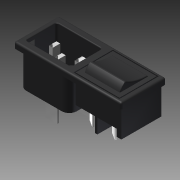
# Autodesk Inventor part: BZM27-Z0000-57B
Saved by Autodesk Inventor 2015 (Build 190159000, 159)
## iProperties
Created: 2013-06-08
Part Number: BZM27-Z0000-57B
Document SubType Name: Modeling
Designer: Estacion4
Density: 1 g/cm^3
Mass: 14.532 g
Surface Area: 93.949 cm^2
Volume: 14.532 cm^3
Material: Generic
Appearance: Rubber - Black - Version 1.1
Author: Estacion4
Autodesk Inventor part; units mm, degrees
ref_plane "YZ Plane" through (0, 0, 0) normal (1, 0, 0) x (0, 1, 0)
ref_plane "XZ Plane" through (0, 0, 0) normal (0, 1, 0) x (-1, 0, 0)
ref_plane "XY Plane" through (0, 0, 0) normal (0, 0, 1) x (1, 0, 0)
sketch "Boceto1" plane through (0, 0, 0) normal (0, 0, 1) x (1, 0, 0)
  line L0 (-28.75, 12) -> (28.75, 12)
  line L1 (28.75, 12) -> (28.75, -12)
  line L2 (28.75, -12) -> (-28.75, -12)
  line L3 (-28.75, -12) -> (-28.75, 12)
  line L4 (-27.45, 10.65) -> (27.45, 10.65)
  line L5 (27.45, 10.65) -> (27.45, -10.65)
  line L6 (27.45, -10.65) -> (-27.45, -10.65)
  line L7 (-27.45, -10.65) -> (-27.45, 10.65)
  point P0 (0, 0)
  point P1 (0, 12)
  point P2 (-28.75, 0)
  point P3 (-27.45, 0)
  point P4 (0, 10.65)
  dimension "d0" = 57.5
  dimension "d1" = 24
  dimension "d2" = 54.9
  dimension "d3" = 21.3
  constraints: 16 end point, 4 midpoint, 4 parallel, 2 horizontal, 2 horizontal alignment, 2 perpendicular, 2 vertical alignment
  measures "d0" distance of L0.start L0.end
  measures "d1" distance of L2.end L0.start
  measures "d2" distance of L4.start L4.end
  measures "d3" distance of L6.end L4.start
extrude "Extrusión1" add sketch "Boceto1" along normal blind 3.2 contours L0 L1 L2 L3 | L4 L5 L6 L7
sketch "Boceto2" plane through (0, 0, 0) normal (0, 0, -1) x (-1, 0, 0)
  line L0 (28.75, -12) -> (28.75, 12) projected
  line L1 (27.45, -10.65) -> (0.45, -10.65)
  line L2 (0.45, -10.65) -> (0.45, 10.65)
  line L3 (0.45, 10.65) -> (27.45, 10.65)
  line L4 (27.45, 10.65) -> (27.45, -10.65)
  line L5 (28.75, 12) -> (-28.75, 12) projected
  line L6 (-28.75, 12) -> (-28.75, -12) projected
  line L7 (-28.75, -12) -> (28.75, -12) projected
  line L8 (28.75, -12) -> (28.75, 12) projected
  point P0 (27.45, 0)
  point P1 (28.75, 0)
  point P2 (27.45, 0)
  dimension "d8" = 27
  dimension "d9" = 21.3
  constraints: 8 end point, 2 midpoint, 2 parallel, 1 coincident, 1 horizontal, 1 horizontal alignment, 1 perpendicular
  measures "d8" distance of L1.start L1.end
  measures "d9" distance of L3.end L1.start
extrude "Extrusión3" add sketch "Boceto2" along normal blind 17.8 contours L1 L2 L3 L4
fillet "Empalme1" radius 4 4 edges at (-27.45, -10.65, -8.9) (-27.45, 10.65, -8.9) (-0.45, 10.65, -8.9) (-0.45, -10.65, -8.9)
sketch "Boceto3" plane through (0, 0, 0) normal (0, 0, -1) x (-1, 0, 0)
  line L0 (-3.05, -10.65) -> (-27.45, -10.65)
  line L1 (-27.45, -10.65) -> (-27.45, 10.65)
  line L2 (-27.45, 10.65) -> (-3.05, 10.65)
  line L3 (-3.05, 10.65) -> (-3.05, -10.65)
  line L4 (-27.45, 10.65) -> (-27.45, -10.65) projected
  line L5 (-27.45, -10.65) -> (27.45, -10.65) projected
  line L6 (27.45, 10.65) -> (-27.45, 10.65) projected
  dimension "d13" = 24.4
  constraints: 8 end point, 2 parallel, 1 horizontal, 1 perpendicular
  measures "d13" distance between parallel lines of L1 L3
extrude "Extrusión4" add sketch "Boceto3" along normal blind 11.2
sketch "Boceto4" plane through (0, 0, -11.2) normal (0, 0, -1) x (-1, 0, 0)
  line L0 (-27.45, 10.65) -> (-3.05, 10.65) projected
  line L1 (-27.45, -10.65) -> (-27.45, 10.65) projected
  line L2 (-3.05, -10.65) -> (-27.45, -10.65) projected
  line L3 (-24.95, -10.65) -> (-24.95, 10.65)
  dimension "d16" = 2.5
  constraints: 2 end point, 2 point on line, 1 perpendicular
  measures "d16" distance between parallel lines of L1 L3
extrude "Extrusión5" add sketch "Boceto4" along normal blind 3.75
sketch "Boceto5" plane through (0, 0, -11.2) normal (0, 0, -1) x (-1, 0, 0)
  line L0 (-3.05, -10.65) -> (-24.95, -10.65) projected
  line L1 (-24.95, 10.65) -> (-3.05, 10.65) projected
  line L2 (-13.375, -10.65) -> (-14.625, -10.65)
  line L3 (-14.625, -10.65) -> (-14.625, 10.65)
  line L4 (-14.625, 10.65) -> (-13.375, 10.65)
  line L5 (-13.375, 10.65) -> (-13.375, -10.65)
  point P0 (-14, -10.65)
  dimension "d19" = 1.25
  constraints: 8 end point, 2 midpoint, 2 parallel, 2 point on line, 1 horizontal, 1 perpendicular
  measures "d19" distance between parallel lines of L3 L5
extrude "Extrusión6" add sketch "Boceto5" along normal blind 7.8
sketch "Boceto6" plane through (0, 0, -11.2) normal (0, 0, -1) x (-1, 0, 0)
  line L0 (-14.625, -10.65) -> (-14.625, 10.65) projected
  line L1 (-24.95, 10.65) -> (-14.625, 10.65) projected
  line L2 (-24.95, 10.65) -> (-24.95, -10.65) projected
  line L3 (-14.625, -10.65) -> (-24.95, -10.65) projected
  line L4 (-5.9821, -6.1326) -> (-9.9328, -8.6786)
  line L5 (-9.9328, -8.6786) -> (-10.3661, -8.0061)
  line L6 (-10.3661, -8.0061) -> (-6.4155, -5.4601)
  line L7 (-6.4155, -5.4601) -> (-5.9821, -6.1326)
  dimension "d22" = 0.8
  dimension "d23" = 4.7
  constraints: 8 end point, 2 parallel, 1 perpendicular
  measures "d22" distance between parallel lines of L6 L4
  measures "d23" distance of L4.start L4.end
extrude "Extrusión7" add sketch "Boceto6" along normal up to surface (7.8 mm away) contours L4 L5 L6 L7
pattern_linear "Patrón rectangular1" count 2 spacing 12 along (1, 0, 0) count 2 spacing 6 along (0, 1, 0) of "Extrusión7"
sketch "Boceto7" plane through (0, 0, -17.8) normal (0, 0, -1) x (-1, 0, 0)
  line L0 (27.45, 6.65) -> (27.45, -6.65) projected
  line L1 (4.45, 10.65) -> (23.45, 10.65) projected
  line L2 (17.1, -6.75) -> (10.8, -6.75)
  line L3 (10.8, -6.75) -> (10.8, -5.75)
  line L4 (10.8, -5.75) -> (17.1, -5.75)
  line L5 (17.1, -5.75) -> (17.1, -6.75)
  line L6 (23.95, 4.75) -> (17.65, 4.75)
  line L7 (17.65, 4.75) -> (17.65, 5.75)
  line L8 (17.65, 5.75) -> (23.95, 5.75)
  line L9 (23.95, 5.75) -> (23.95, 4.75)
  line L10 (10.25, 4.75) -> (3.95, 4.75)
  line L11 (3.95, 4.75) -> (3.95, 5.75)
  line L12 (3.95, 5.75) -> (10.25, 5.75)
  line L13 (10.25, 5.75) -> (10.25, 4.75)
  line L14 (17.65, 5.75) -> (10.25, 5.75) construction
  line L15 (13.95, -5.75) -> (13.95, 5.75) construction
  point P0 (13.95, 0)
  point P1 (27.45, 0)
  point P2 (13.95, 10.65)
  dimension "d32" = 12.5
  dimension "d33" = 20
  dimension "d34" = 1
  dimension "d35" = 6.3
  constraints: 28 end point, 10 parallel, 5 midpoint, 5 perpendicular, 3 horizontal, 2 horizontal alignment, 1 vertical alignment
  measures "d32" distance between parallel lines of L8 L2
  measures "d33" distance between parallel lines of L11 L9
  measures "d34" distance of L4.end L2.start
  measures "d35" distance of L2.start L2.end
extrude "Extrusión8" add sketch "Boceto7" along normal blind 11
sketch "Boceto8" plane through (0, 0, 3.2) normal (0, 0, 1) x (1, 0, 0)
  line L0 (-0.45, -6.65) -> (-0.45, 6.65) projected
  arc A0 (-4.45, -10.65) -> (-0.45, -6.65) centre (-4.45, -6.65) ccw projected
  line L1 (-23.45, -10.65) -> (-4.45, -10.65) projected
  arc A1 (-27.45, -6.65) -> (-23.45, -10.65) centre (-23.45, -6.65) ccw projected
  line L2 (-27.45, 6.65) -> (-27.45, -6.65) projected
  arc A2 (-23.45, 10.65) -> (-27.45, 6.65) centre (-23.45, 6.65) ccw projected
  line L3 (-4.45, 10.65) -> (-23.45, 10.65) projected
  arc A3 (-0.45, 6.65) -> (-4.45, 10.65) centre (-4.45, 6.65) ccw projected
  line L4 (-1.85, 8.2) -> (-26.05, 8.2)
  line L5 (-26.05, 8.2) -> (-26.05, -3.6)
  line L6 (-26.05, -3.6) -> (-21.45, -8.2)
  line L7 (-21.45, -8.2) -> (-6.45, -8.2)
  line L8 (-6.45, -8.2) -> (-1.85, -3.6)
  line L9 (-1.85, -3.6) -> (-1.85, 8.2)
  line L10 (-13.95, -8.2) -> (-13.95, 8.2) construction
  point P0 (-13.95, 10.65)
  point P1 (-13.95, 0)
  point P2 (-27.45, 0)
  dimension "d38" = 24.2
  dimension "d39" = 16.4
  dimension "d40" = 15
  dimension "d41" = 90
  constraints: 14 end point, 5 midpoint, 4 parallel, 2 perpendicular, 2 vertical alignment, 1 horizontal alignment
  measures "d38" distance of L4.start L4.end
  measures "d39" distance between parallel lines of L4 L7
  measures "d40" distance of L6.end L7.end
  measures "d41" angle of L6 L8
extrude "Extrusión9" cut sketch "Boceto8" against normal blind 19 contours L9 L8 L7 L6 L5 L4
sketch "Boceto9" plane through (0, 0, 3.2) normal (0, 0, 1) x (1, 0, 0)
  line L0 (-1.85, -3.6) -> (-6.45, -8.2) projected
  line L1 (-21.45, -8.2) -> (-26.05, -3.6) projected
  line L2 (28.75, -12) -> (-28.75, -12) projected
  line L3 (-1.85, -3.6) -> (-1.85, -8.2)
  line L4 (-1.85, -8.2) -> (-6.45, -8.2)
  line L5 (-21.45, -8.2) -> (-26.05, -8.2)
  line L6 (-26.05, -8.2) -> (-26.05, -3.6)
  constraints: 8 end point, 3 perpendicular, 1 collinear
extrude "Extrusión10" cut sketch "Boceto9" against normal blind 2
fillet "Empalme2" radius 1 4 edges at (-26.05, -8.2, 2.2) (-1.85, -8.2, 2.2) (-1.85, 8.2, -6.3) (-26.05, 8.2, -6.3)
fillet "Empalme3" radius 0.5 8 edges at (-13.95, -8.2, 3.2) (-25.7571, -7.9071, 3.2) (-26.05, 0, 3.2) (-25.7571, 7.9071, 3.2) (-13.95, 8.2, 3.2) (-2.1429, 7.9071, 3.2) (-1.85, 0, 3.2) (-2.1429, -7.9071, 3.2)
sketch "Boceto10" plane through (0, 0, -15.8) normal (0, 0, 1) x (1, 0, 0)
  line L0 (-2.85, 8.2) -> (-25.05, 8.2) projected
  line L1 (-12.95, -4.1) -> (-14.95, -4.1)
  line L2 (-14.95, -4.1) -> (-14.95, -0.1)
  line L3 (-14.95, -0.1) -> (-12.95, -0.1)
  line L4 (-12.95, -0.1) -> (-12.95, -4.1)
  line L5 (-6.05, -0.1) -> (-8.05, -0.1)
  line L6 (-8.05, -0.1) -> (-8.05, 3.9)
  line L7 (-8.05, 3.9) -> (-6.05, 3.9)
  line L8 (-6.05, 3.9) -> (-6.05, -0.1)
  line L9 (-19.85, -0.1) -> (-21.85, -0.1)
  line L10 (-21.85, -0.1) -> (-21.85, 3.9)
  line L11 (-21.85, 3.9) -> (-19.85, 3.9)
  line L12 (-19.85, 3.9) -> (-19.85, -0.1)
  line L13 (-8.05, 3.9) -> (-19.85, 3.9) construction
  line L14 (-25.05, 8.2) -> (-2.85, 8.2) construction
  point P0 (-13.95, -0.1)
  point P1 (-13.95, 3.9)
  point P2 (-13.95, -4.1)
  point P3 (-13.95, 8.2)
  dimension "d48" = 11.8
  dimension "d49" = 2
  dimension "d50" = 4
  dimension "d51" = 4.3
  constraints: 26 end point, 6 parallel, 4 equal length, 4 midpoint, 4 perpendicular, 3 horizontal, 2 horizontal alignment, 2 vertical alignment
  measures "d48" distance of L6.end L11.end
  measures "d49" distance between parallel lines of L2 L4
  measures "d50" distance of L1.end L2.end
  measures "d51" distance between parallel lines of L7 L0
extrude "Extrusión11" add sketch "Boceto10" along normal blind 15.2
fillet "Empalme4" radius 1 4 edges at (28.75, -12, 1.6) (28.75, 12, 1.6) (-28.75, 12, 1.6) (-28.75, -12, 1.6)
fillet "Empalme5" radius 1 8 edges at (0, -12, 3.2) (-28.4571, -11.7071, 3.2) (-28.75, 0, 3.2) (-28.4571, 11.7071, 3.2) (0, 12, 3.2) (28.4571, 11.7071, 3.2) (28.75, 0, 3.2) (28.4571, -11.7071, 3.2)
chamfer "Chaflán1" distance 0.75 angle 45 12 edges at (-7.05, -0.1, -0.6) (-8.05, 1.9, -0.6) (-7.05, 3.9, -0.6) (-6.05, 1.9, -0.6) (-13.95, -4.1, -0.6) (-14.95, -2.1, -0.6) (-13.95, -0.1, -0.6) (-12.95, -2.1, -0.6) (-20.85, -0.1, -0.6) (-19.85, 1.9, -0.6) (-21.85, 1.9, -0.6) (-20.85, 3.9, -0.6)
sketch "Boceto11" plane through (0, 0, 3.2) normal (0, 0, 1) x (1, 0, 0)
  line L0 (27.75, 11) -> (27.75, -11) projected
  line L1 (26.25, -10.5) -> (1.75, -10.5)
  line L2 (1.75, -10.5) -> (1.75, 10.5)
  line L3 (1.75, 10.5) -> (26.25, 10.5)
  line L4 (26.25, 10.5) -> (26.25, -10.5)
  line L5 (28.75, -11) -> (28.75, 11) projected
  line L6 (2.25, -10) -> (25.75, -10)
  line L7 (25.75, -10) -> (25.75, 10)
  line L8 (25.75, 10) -> (2.25, 10)
  line L9 (2.25, 10) -> (2.25, -10)
  point P0 (26.25, 0)
  point P1 (27.75, 0)
  dimension "d59" = 24.5
  dimension "d60" = 21
  dimension "d61" = 2.5
  dimension "d62" = 0.5
  constraints: 16 end point, 4 parallel, 2 midpoint, 2 perpendicular, 1 horizontal, 1 horizontal alignment, 3 other
  measures "d59" distance of L1.start L1.end
  measures "d60" distance of L3.end L1.start
  measures "d61" distance between parallel lines of L5 L4
  measures "d62" distance between parallel lines of L1 L6
extrude "Extrusión12" cut sketch "Boceto11" against normal blind 1
sketch "Boceto12" plane through (0, 0, 3.2) normal (0, 0, 1) x (1, 0, 0)
  line L0 (25.75, -10) -> (25.75, 10) projected
  line L1 (25.75, 10) -> (2.25, 10) projected
  line L2 (4.5, 7.5) -> (23.5, 7.5)
  line L3 (23.5, 7.5) -> (23.5, -7.5)
  line L4 (23.5, -7.5) -> (4.5, -7.5)
  line L5 (4.5, -7.5) -> (4.5, 7.5)
  point P0 (23.5, 0)
  point P1 (25.75, 0)
  point P2 (14, 7.5)
  point P3 (14, 10)
  dimension "d65" = 19
  dimension "d66" = 15
  constraints: 8 end point, 4 midpoint, 2 parallel, 1 horizontal, 1 horizontal alignment, 1 perpendicular, 1 vertical alignment
  measures "d65" distance of L2.start L2.end
  measures "d66" distance of L2.end L3.end
extrude "Extrusión13" add sketch "Boceto12" along normal blind 3.5
sketch "Boceto13" plane through (4.5, -7.5, 3.2) normal (-1, 0, 0) x (0, 0, 1)
  line L0 (3.5, 0) -> (3.5, 15) projected
  line L1 (0, 15) -> (3.5, 15) projected
  line L2 (0, 0) -> (3.5, 0) projected
  arc A0 (0.4945, 15) -> (3.5, 3.2828) centre (25.0341, 15.0504) ccw
  arc A1 (0, 0) -> (3.5, 2.6389) centre (-3.2803, 7.9912) ccw
  constraints: 4 point on circle, 3 point on line, 2 centre point
extrude "Extrusión14" cut sketch "Boceto13" against normal through all
fillet "Empalme6" radius 0.5 9 edges at (4.5, 1.4533, 4.4639) (4.5, -6.4062, 5.1202) (14, -4.8611, 6.7) (14, -4.2172, 6.7) (14, 7.5, 3.6945) (23.5, 1.4533, 4.4639) (23.5, -6.4062, 5.1202) (23.5, -4.5392, 6.7) (4.5, -4.5392, 6.7)
body "Solid1"
